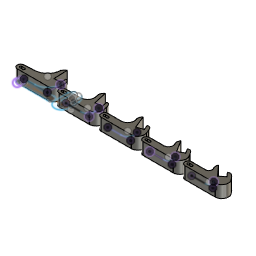
2020_09_18_Phone Holder from left over v3 (Autodesk Fusion 360 design; units mm, degrees)
Autodesk Fusion 360 part; units mm, degrees
note: some values were not read from the file. Set by a fixed rule: which sketch regions a step uses.
sketch "PhoneHolderShape" plane through (0, 0, 0) normal (0, 0, 1) x (1, 0, 0)
  line L0 (-21.1586, 2.1753) -> (23.8414, 2.1753)
  arc A0 (23.8414, 2.1753) -> (23.8414, 12.1753) centre (23.8414, 7.1753) ccw
  line L1 (23.8414, 12.1753) -> (-21.1586, 12.1753)
  arc A1 (-21.1586, 12.1753) -> (-21.1586, 2.1753) centre (-21.1586, 7.1753) ccw
  line L2 (-21.1586, 7.1753) -> (23.8414, 7.1753) construction
  line L3 (23.8414, 7.1753) -> (39.8414, 7.1753) construction
  line L4 (49.8402, 7.3307) -> (49.5915, 23.3287)
  line L5 (29.5297, 27.1497) -> (29.8426, 7.0198)
  arc A2 (29.8426, 7.0198) -> (49.8402, 7.3307) centre (39.8414, 7.1753) ccw
  line L6 (39.8414, 7.1753) -> (39.5927, 23.1733) construction
  line L7 (39.8414, 7.1753) -> (53.8328, 7.3927) construction
  line L8 (34.1604, 32.531) -> (34.958, 12.1753)
  line L9 (34.958, 12.1753) -> (44.958, 12.1753)
  line L10 (44.958, 12.1753) -> (44.1788, 32.0597)
  line L11 (42.2666, 29.5183) -> (34.958, 12.1753) construction
  line L12 (37.2318, 28.0129) -> (44.958, 12.1753) construction
  arc A3 (49.5915, 23.3287) -> (44.1788, 32.0597) centre (39.5927, 23.1733) ccw
  arc A4 (34.1604, 32.531) -> (29.5297, 27.1497) centre (39.5927, 23.1733) ccw
  line L13 (-21.1586, 5.6703) -> (-16.1586, 5.6703)
  arc A5 (-16.1586, 5.6703) -> (-16.1586, 8.6803) centre (-16.1586, 7.1753) ccw
  line L14 (-16.1586, 8.6803) -> (-21.1586, 8.6803)
  arc A6 (-21.1586, 8.6803) -> (-21.1586, 5.6703) centre (-21.1586, 7.1753) ccw
  line L15 (-21.1586, 7.1753) -> (-16.1586, 7.1753) construction
  arc A7 (-21.1586, 8.6803) -> (-21.1586, 5.6703) centre (-21.1586, 7.1753) ccw
  spline S0 degree 5 poles (49.7649, 12.1753) (49.7575, 12.469) (49.7348, 13.0453) (49.677, 13.8757) (49.5514, 14.9138) (49.3079, 16.0881) (48.969, 17.1264) (48.5251, 18.0151) (47.9682, 18.7425) (47.2975, 19.3077) (46.5197, 19.7201) (45.8176, 19.9363) (45.2488, 20.0382) (44.8511, 20.0798) (44.6477, 20.0941) knots 0 0 0 0 0 0 0.1 0.2 0.3 0.4 0.5 0.6 0.7 0.8 0.9 1 1 1 1 1 1
  point P0 (39.5927, 23.1733)
  point P1 (48.2494, 18.3364)
  dimension "d1" = 10
  dimension "d7" = 3.01
  dimension "d8" = 16
  dimension "d9" = 16
  dimension "d10" = 90
  dimension "d11" = 20
  dimension "d12" = 10
  dimension "d13" = 16
  dimension "d28" = 45
  constraint tangent L0 A0
  constraint tangent A0 L1
  constraint parallel L0 L1
  constraint tangent L1 A1
  constraint tangent L0 A1
  constraint horizontal L2
  constraint concentric A1 A7
  constraint coincident A0.centre L2.end
  constraint parallel L2 L3
  constraint tangent L4 A3
  constraint tangent L5 A3
  constraint parallel L4 L5
  constraint tangent L5 A2
  constraint tangent L4 A2
  constraint coincident L3.end A2.centre
  constraint parallel L8 L10
  constraint coincident L11 P0
  constraint coincident L12 P0
  constraint coincident P0 L6.end
  constraint concentric A3 A4
  constraint tangent L13 A5
  constraint tangent A5 L14
  constraint parallel L13 L14
  constraint tangent L14 A6
  constraint tangent L13 A6
  constraint parallel L2 L15
  constraint coincident A1.centre L2.start
  constraint coincident L4 S0.start
  constraint coincident L10 S0.end
  measures "d1" diameter of A0
  measures "d7" diameter of A7
  measures "d8" distance of A0.centre L3.end
  measures "d9" distance of L3.end P0
  measures "d10" angle of L6 L7
  measures "d11" diameter of A3
  measures "d12" distance of L8.end L9.end
  measures "d13" distance of L12.start L8.end
  measures "d28" distance of A0.end L1.end
sketch "Wood Pro 3018" plane through (0, 0, 0) normal (0, 0, 1) x (1, 0, 0)
  line L0 (0, 0) -> (250, 0)
  line L1 (250, 0) -> (250, 150)
  line L2 (250, 150) -> (0, 150)
  line L3 (0, 150) -> (0, 0)
  dimension "d2" = 250
  dimension "d3" = 150
  constraint horizontal L0
  constraint vertical L1
  constraint horizontal L2
  constraint vertical L3
  constraint coincident L0.start L3.end
  measures "d2" distance of L0.start L0.end
  measures "d3" distance of L0.start L2.end
extrude "Extrude1" add sketch "Wood Pro 3018" along normal blind 18 makes body 1
extrude "Extrude2" add sketch "PhoneHolderShape" along normal blind 18 separate body makes body 2 at (45.3968, -1.1397, 6) makes body 3 at (8.8414, 12.1753, 12)
extrude "Extrude4" cut sketch "PhoneHolderShape" along normal blind 18 contours L4 L10 A3 S0 bodies 2
pattern_linear "R-Pattern1" count 5 spacing 62.5 along (1, 0, 0) of bodies 3 makes body 4 at (71.3414, 12.1753, 12) makes body 5 at (133.8414, 12.1753, 12) makes body 6 at (196.3414, 12.1753, 12) makes body 7 at (258.8414, 12.1753, 12)
move_body "Move1" bodies 2 to x (1, 0, 0) y (0, 1, 0) z (0, 0, 1) at (-16.1554, 4.9988, 0)
pattern_linear "R-Pattern2" count 5 spacing 62.5 along (1, 0, 0) of bodies 2 makes body 8 at (79.6865, 4.5743, 12) makes body 9 at (157.2989, 7.0929, 12) makes body 10 at (219.7989, 7.0929, 12) makes body 11 at (269.7153, 2.9962, 12)
move_body "Move2" bodies 8 to x (0.984808, 0.173648, 0) y (-0.173648, 0.984808, 0) z (0, 0, 1) at (3.4234, -14.7811, 0)
move_body "Move3" bodies 9 to x (0.939693, 0.34202, 0) y (-0.34202, 0.939693, 0) z (0, 0, 1) at (13.1306, -50.1194, 0)
move_body "Move4" bodies 10 to x (0.866025, 0.5, 0) y (-0.5, 0.866025, 0) z (0, 0, 1) at (34.3806, -103.962, 0)
move_body "Move5" bodies 11 to x (0.766044, 0.642788, 0) y (-0.642788, 0.766044, 0) z (0, 0, 1) at (71.8557, -173.0738, 0)
combine "Combine1" operation add target body 2 tool bodies 3
combine "Combine2" operation add target body 8 tool bodies 4
combine "Combine3" operation add target body 9 tool bodies 5
combine "Combine4" operation add target body 10 tool bodies 6
combine "Combine5" operation add target body 11 tool bodies 7
sketch "Corners" plane through (0, 0, 0) normal (0, 0, 1) x (1, 0, 0)
  arc A0 (-21.1586, 12.1753) -> (-21.1586, 2.1753) centre (-21.1586, 7.1753) ccw
  line L0 (-21.1586, 12.1753) -> (-5.4542, 13.11)
  line L1 (13.3743, 32.1485) -> (13.6848, 12.1753)
  line L2 (13.3551, 33.3855) -> (13.3743, 32.1485)
  line L3 (72.5624, 30.0545) -> (76.0024, 12.1753)
  line L4 (72.5624, 30.0545) -> (73.6209, 23.8594)
  line L5 (132.1645, 27.4171) -> (137.9819, 12.1753)
  line L6 (132.1645, 27.4171) -> (132.8042, 25.7411)
  line L7 (137.9819, 12.1753) -> (103.8414, 12.1753)
  line L8 (123.4616, 12.1753) -> (103.8414, 12.1753)
  line L9 (63.7637, 12.1753) -> (41.3414, 12.1753)
  line L10 (192.2686, 24.3166) -> (199.5323, 12.1753)
  line L11 (192.2686, 24.3166) -> (193.1944, 22.769)
  arc A1 (-5.4542, 13.11) -> (13.3551, 33.3855) centre (-6.6425, 33.0747) ccw
  arc A2 (63.7637, 12.1753) -> (73.6209, 23.8594) centre (63.7637, 22.1753) ccw
  arc A3 (123.4616, 12.1753) -> (132.8042, 25.7411) centre (123.4616, 22.1753) ccw
  line L12 (199.5323, 12.1753) -> (166.3414, 12.1753)
  line L13 (187.1874, 12.1753) -> (166.3414, 12.1753)
  line L14 (228.8414, 12.1753) -> (249.513, 12.1753)
  line L15 (252.9474, 20.8472) -> (260.4568, 12.1753)
  line L16 (253.2928, 20.4483) -> (252.9474, 20.8472)
  arc A4 (187.1874, 12.1753) -> (193.1944, 22.769) centre (187.1874, 19.1753) ccw
  arc A5 (249.513, 12.1753) -> (253.2928, 20.4483) centre (249.513, 17.1753) ccw
  line L17 (-21.1586, 12.1753) -> (13.6848, 12.1753)
  line L18 (41.3414, 12.1753) -> (76.0024, 12.1753)
  line L19 (228.8414, 12.1753) -> (260.4568, 12.1753)
  line L20 (199.5323, 12.1753) -> (166.3414, 12.1753)
  line L21 (192.2686, 24.3166) -> (199.5323, 12.1753)
  line L22 (252.9474, 20.8472) -> (260.4568, 12.1753)
  line L23 (137.9819, 12.1753) -> (132.1645, 27.4171)
  line L24 (137.9819, 12.1753) -> (103.8414, 12.1753)
  line L25 (72.5624, 30.0545) -> (76.0024, 12.1753)
  line L26 (13.6848, 12.1753) -> (13.3743, 32.1485)
  point P0 (-21.1586, 12.1753)
  point P1 (13.6848, 12.1753)
  point P2 (13.3743, 32.1485)
  point P3 (72.5624, 30.0545)
  point P4 (76.0024, 12.1753)
  point P5 (132.1645, 27.4171)
  point P6 (137.9819, 12.1753)
  point P7 (103.8414, 12.1753)
  point P8 (41.3414, 12.1753)
  point P9 (192.2686, 24.3166)
  point P10 (199.5323, 12.1753)
  point P11 (166.3414, 12.1753)
  point P12 (228.8414, 12.1753)
  point P13 (260.4568, 12.1753)
  point P14 (252.9474, 20.8472)
  dimension "d32" = 20
  dimension "d33" = 10
  dimension "d34" = 10
  dimension "d35" = 7
  dimension "d36" = 5
  constraint coincident P0 A0.start
  constraint coincident P2 L1.start
  constraint coincident P3 L3.start
  constraint coincident P5 L5.start
  constraint coincident P7 L7.end
  constraint coincident P8 L9.end
  constraint coincident P9 L10.start
  constraint tangent L2 A1
  constraint tangent L0 A1
  constraint tangent L4 A2
  constraint tangent L9 A2
  constraint tangent L8 A3
  constraint tangent L6 A3
  constraint coincident P11 L12.end
  constraint coincident P12 L14.start
  constraint coincident P14 L15.start
  constraint tangent L13 A4
  constraint tangent L11 A4
  constraint tangent L14 A5
  constraint tangent L16 A5
  constraint coincident P1 L1.end
  constraint coincident P4 L3.end
  constraint parallel L9 L18
  constraint coincident P13 L15.end
  constraint parallel L14 L19
  constraint coincident P10 L10.end
  constraint parallel L13 L20
  constraint coincident P6 L5.end
  constraint parallel L2 L26
  measures "d32" radius of A1
  measures "d33" radius of A2
  measures "d34" radius of A3
  measures "d35" radius of A4
  measures "d36" radius of A5
extrude "Extrude3" add sketch "Corners" along normal blind 18 bodies 2 8 9 10 11
hidden bodies 1
equation "WoodHeight = 18 mm"
equation "d5 = WoodHeight"
equation "d9 = HolderHeight"
equation "d11 = PhoneHeight + 10 mm"
equation "d12 = PhoneHeight"
equation "d14 = WoodHeight"
equation "d28 = LenghBase"
equation "LenghBase = 45 mm"
equation "PhoneHeight = 10 mm"
equation "HolderHeight = 16 mm"
equation "d37 = WoodHeight"
equation "d39 = WoodHeight"
named bodies: "Wood Pro 3018"
